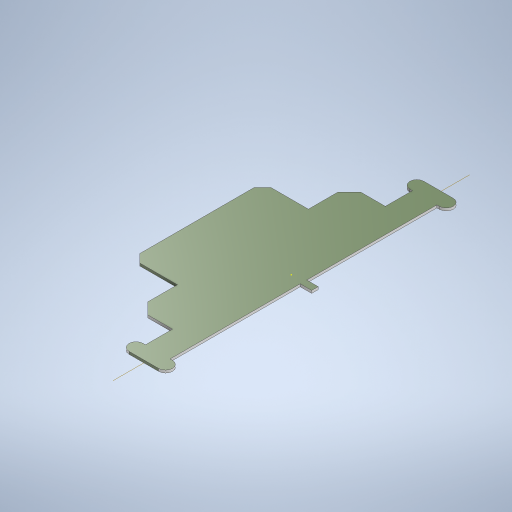
# Autodesk Inventor part: linefollower_chassy_model
Saved by Autodesk Inventor 2024 (Build 280153000, 153)
## iProperties
Created: 2024-02-06
Part Number: linefollower_chassy_model
Material: Generic
Document SubType Name: Modeling
Designer: kamil
Density: 1 g/cm^3
Appearance: Default
Author: kamil
Autodesk Inventor part; units mm, degrees
ref_plane "YZ Plane" through (0, 0, 0) normal (1, 0, 0) x (0, 1, 0)
ref_plane "XZ Plane" through (0, 0, 0) normal (0, 1, 0) x (-1, 0, 0)
ref_plane "XY Plane" through (0, 0, 0) normal (0, 0, 1) x (1, 0, 0)
sketch "Sketch1" plane through (0, 0, 0) normal (0, 1, 0) x (-1, 0, 0)
  line L0 (7.5, 90) -> (-7.5, 90)
  line L1 (-7.5, -90) -> (7.505, -90)
  line L2 (7.5, -86.9) -> (7.5, -84.6)
  line L3 (29.5, 40) -> (52.5, 40)
  line L4 (57.5, 35) -> (57.5, -35)
  line L5 (52.5, -40) -> (29.5, -40)
  line L6 (-7.5, 2) -> (-14.5, 2)
  line L7 (-14.5, 2) -> (-14.5, -2)
  line L8 (-14.5, -2) -> (-7.5, -2)
  circle A0 centre (-12.5, 0) radius 1.5
  line L9 (52.5, -40) -> (57.5, -35)
  line L10 (52.5, 40) -> (57.5, 35)
  line L11 (7.505, -90) -> (9.005, -90)
  line L12 (7.5, -81.5) -> (9.01, -81.5)
  arc A1 (9.005, -90) -> (9.01, -81.5) centre (9.0075, -85.75) ccw
  line L13 (7.5, -84.6) -> (9, -84.6)
  line L14 (7.5, -86.9) -> (9, -86.9)
  arc A2 (9, -86.9) -> (9, -84.6) centre (9, -85.75) ccw
  line L15 (-7.5, -90) -> (-9, -90)
  line L16 (-7.5, -81.5) -> (-9.01, -81.5)
  arc A3 (-9.01, -81.5) -> (-9, -90) centre (-9.005, -85.75) ccw
  line L17 (-7.5, -84.6) -> (-9, -84.6)
  line L18 (-7.5, -86.9) -> (-9, -86.9)
  arc A4 (-9, -84.6) -> (-9, -86.9) centre (-9, -85.75) ccw
  arc A5 (9.01, 81.5) -> (9.005, 90) centre (9.005, 85.75) ccw
  arc A6 (9, 84.6) -> (9, 86.9) centre (9, 85.75) ccw
  arc A7 (-9, 86.9) -> (-9, 84.6) centre (-9, 85.75) ccw
  arc A8 (-9, 90) -> (-9.01, 81.5) centre (-9.005, 85.75) ccw
  line L19 (9.005, 90) -> (7.5, 90)
  line L20 (9.01, 81.5) -> (7.5, 81.5)
  line L21 (-9, 90) -> (-7.5, 90)
  line L22 (-9.01, 81.5) -> (-7.5, 81.5)
  line L23 (7.5, 65) -> (22.5, 65)
  line L24 (22.5, -65) -> (7.5, -65)
  line L25 (7.5, -65) -> (7.5, -40)
  line L26 (29.5, 58) -> (22.5, 65)
  line L27 (29.5, -58) -> (22.5, -65)
  line L28 (9, 84.6) -> (7.5, 84.6)
  line L29 (9, 86.9) -> (7.5, 86.9)
  line L30 (-9, 86.9) -> (-7.5, 86.9)
  line L31 (-9, 84.6) -> (-7.5, 84.6)
  circle A9 centre (51.5, 0) radius 1.5
  line L32 (7.5, 84.6) -> (7.5, 86.9)
  line L33 (-7.5, 86.9) -> (-7.5, 84.6)
  line L34 (7.5, 65) -> (7.5, 81.5)
  line L35 (29.5, 58) -> (29.5, 40)
  line L36 (29.5, -40) -> (29.5, -58)
  line L37 (-7.5, 81.5) -> (-7.5, 2)
  line L38 (7.5, -86.9) -> (7.5, -84.6)
  line L39 (7.5, -81.5) -> (7.5, -65)
  line L40 (-7.5, -2) -> (-7.5, -81.5)
  line L41 (-7.5, -84.6) -> (-7.5, -86.9)
  point P0 (0, 0)
  point P1 (0, 0)
  point P2 (0, 0)
  point P3 (57.5, -40)
  point P4 (57.5, 40)
  point P5 (57.5, 0)
  point P6 (15, 0)
  point P7 (-11, -2)
  point P8 (-14.5, 0)
  point P9 (-7.5, 0)
  point P10 (8.255, -90)
  point P11 (8.255, -81.5)
  point P12 (-8.25, -90)
  point P13 (-8.255, -81.5)
  point P14 (8.25, 90)
  point P15 (8.255, 81.5)
  point P16 (-8.25, 90)
  point P17 (-8.255, 81.5)
  point P18 (29.5, -65)
  point P19 (29.5, 65)
  point P20 (29.5, 0)
  point P21 (0, 0)
  point P22 (7.5, 85.75)
  dimension "d5" = 50
  dimension "d6" = 80
  dimension "d7" = 3
  dimension "d8" = 4
  dimension "d10" = 5
  dimension "d11" = 5
  dimension "d12" = 5
  dimension "d13" = 5
  dimension "d14" = 5
  dimension "d17" = 180
  dimension "d18" = 1.5
  dimension "d19" = 1.51
  dimension "d20" = 8.5
  dimension "d21" = 1.5
  dimension "d22" = 3.1
  dimension "d23" = 1.5
  dimension "d24" = 2.3
  dimension "d26" = 130
  dimension "d27" = 22
  dimension "d28" = 7
  dimension "d29" = 7
  dimension "d30" = 7
  dimension "d31" = 7
  dimension "d32" = 3
  dimension "d33" = 6
  dimension "d34" = 40
  dimension "d35" = 1.5
  dimension "d36" = 4.25
  dimension "d37" = 1.15
  dimension "d38" = 25
  dimension "d39" = 23
  dimension "d40" = 130
  constraints: 84 end point, 26 perpendicular, 23 parallel, 16 point on circle, 10 centre point, 8 point on line, 6 horizontal, 6 midpoint, 3 horizontal alignment, 1 coincident, 1 collinear
  measures "d5" distance of L25.end point (57.5, -40)
  measures "d6" distance of point (57.5, 40) point (57.5, -40)
  measures "d7" diameter of A0
  measures "d8" distance from line of point (-11, -2) L6
  measures "d10" distance of point (-7.5, 0) A0.centre
  measures "d11" distance of L5.start point (57.5, -40)
  measures "d12" distance of L4.end point (57.5, -40)
  measures "d13" distance of L3.end point (57.5, 40)
  measures "d14" distance of L4.start point (57.5, 40)
  measures "d17" distance of L0.end L1.start
  measures "d18" distance of L1.end L11.end
  measures "d19" distance of L12.start L12.end
  measures "d20" distance of point (8.255, -90) point (8.255, -81.5)
  measures "d21" distance of L2.end L13.end
  measures "d22" distance between parallel lines of L13 L12
  measures "d23" distance of L2.start L14.end
  measures "d24" distance between parallel lines of L14 L13
  measures "d26" distance of point (29.5, 65) point (29.5, -65)
  measures "d27" distance of L24.end point (29.5, -65)
  measures "d28" distance of L26.start point (29.5, 65)
  measures "d29" distance of L23.end point (29.5, 65)
  measures "d30" distance of L27.start point (29.5, -65)
  measures "d31" distance of L24.start point (29.5, -65)
  measures "d32" diameter of A9
  measures "d33" distance from line of A9.centre L4
  measures "d34" distance from line of L3 A9.centre
  measures "d35" distance from line of L32 A6.centre
  measures "d36" distance from line of L0 A6.centre
  measures "d37" distance from line of point (7.5, 85.75) L29
  measures "d38" distance between parallel lines of L3 L23
  measures "d39" distance of L3.start L3.end
  measures "d40" distance between parallel lines of L24 L23
extrude "Extrusion1" add sketch "Sketch1" along normal blind 1.57 contours L19 A5 L20 L34 L23 L26 L35 L3 L10 L4 L9 L5 L36 L27 L24 L39 L12 A1 L11 L1 L15 A3 L16 L40 L8 L7 L6 L37 L22 A8 L21 L0 | L2 L13 A2 L14 | A0 | L41 L18 A4 L17 | L28 L32 L29 A6 | L30 L33 L31 A7 | A9
sketch "Sketch2" plane through (0, 1.57, 0) normal (0, 1, 0) x (1, 0, 0)
  point P0 (0, 0)
equation "\"d12\" = d11"
equation "\"d13\" = d11"
equation "\"d14\" = d13"
equation "\"d29\" = d28"
equation "\"d30\" = d28"
equation "\"d31\" = d30"
body "Solid1"
